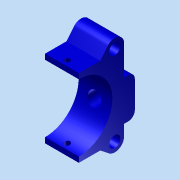
# Autodesk Inventor part: Axle Housing - Front - Custom
Saved by Autodesk Inventor 2012 (Build 160160000, 160)
## iProperties
Created: 2011-09-22
Part Number: Axle Housing - Front - Custom
Document SubType Name: Modeling
Designer: dgitz
Density: 1 g/cm^3
Material: Default
Author: dgitz
Autodesk Inventor part; units mm, degrees
ref_plane "YZ Plane" through (0, 0, 0) normal (1, 0, 0) x (0, 1, 0)
ref_plane "XZ Plane" through (0, 0, 0) normal (0, 1, 0) x (-1, 0, 0)
ref_plane "XY Plane" through (0, 0, 0) normal (0, 0, 1) x (1, 0, 0)
sketch "Sketch2" plane through (0, 0, 0) normal (1, 0, 0) x (0, 1, 0)
  circle A0 centre (100.6118, 121.1829) radius 2.667
  circle A1 centre (62.5118, 121.1829) radius 2.667
  line L0 (100.6118, 121.1829) -> (62.5118, 121.1829) construction
  arc A2 (100.6118, 116.7379) -> (103.3814, 124.6597) centre (100.6118, 121.1829) ccw
  arc A3 (59.0351, 123.9525) -> (62.5118, 116.7379) centre (62.5118, 121.1829) ccw
  line L1 (100.6118, 116.7379) -> (86.6418, 116.7379)
  line L2 (62.5118, 116.7379) -> (67.5918, 116.7379)
  line L3 (67.5918, 116.7379) -> (67.5918, 114.8329)
  line L4 (70.7668, 111.6579) -> (83.4668, 111.6579)
  line L5 (86.6418, 114.8329) -> (86.6418, 116.7379)
  arc A4 (64.8377, 138.2082) -> (96.5877, 138.2082) centre (80.7127, 138.2082) ccw
  line L6 (77.1168, 111.6579) -> (77.1168, 163.1454) construction
  line L7 (99.1277, 138.2082) -> (96.5877, 138.2082)
  line L8 (64.8377, 138.2082) -> (62.2977, 138.2082)
  line L9 (99.1277, 138.2082) -> (99.1277, 128.0482)
  line L10 (99.1277, 128.0482) -> (103.3814, 124.6597)
  line L11 (62.2977, 138.2082) -> (62.2977, 128.0482)
  line L12 (62.2977, 128.0482) -> (59.0351, 123.9525)
  line L13 (99.1277, 128.0482) -> (62.2977, 128.0482) construction
  arc A5 (83.4668, 111.6579) -> (86.6418, 114.8329) centre (83.4668, 114.8329) ccw
  arc A6 (67.5918, 114.8329) -> (70.7668, 111.6579) centre (70.7668, 114.8329) ccw
  point P0 (0, 0)
  point P1 (67.5918, 111.6579)
  point P2 (86.6418, 111.6579)
  dimension "d0" = 5.334
  dimension "d1" = 5.334
  dimension "d2" = 38.1
  dimension "d3" = 8.89
  dimension "d4" = 8.89
  dimension "d7" = 31.75
  dimension "d8" = 9.525
  dimension "d9" = 13.97
  dimension "d10" = 5.08
  dimension "d11" = 2.54
  dimension "d12" = 2.54
  dimension "d13" = 10.16
  dimension "d24" = 3.175
  constraints: 28 end point, 10 point on circle, 8 perpendicular, 8 tangent, 7 centre point, 5 point on line, 2 coincident, 2 horizontal, 2 vertical, 1 collinear, 1 equal radius, 1 midpoint, 1 parallel
  measures "d0" diameter of A0
  measures "d1" diameter of A1
  measures "d2" distance of L0.end L0.start
  measures "d3" diameter of A2
  measures "d4" diameter of A3
  measures "d7" diameter of A4
  measures "d8" distance from line of L4 L0.start
  measures "d9" distance from line of L5 L0.start
  measures "d10" distance from line of L3 L0.end
  measures "d11" distance of L7.end L7.start
  measures "d12" distance of L8.start L8.end
  measures "d13" distance from line of L9.end L7
  measures "d24" radius of A5
extrude "Extrusion1" add sketch "Sketch2" along normal mid plane 16.002
sketch "Sketch3" plane through (-8.001, 99.1277, 128.0482) normal (0, 1, 0) x (1, 0, 0)
  line L0 (0, 0) -> (0, -10.16) projected
  line L1 (0, -10.16) -> (16.002, -10.16) projected
  circle A0 centre (8.001, -7.62) radius 1.27
  point P0 (8.001, 128.0482)
  dimension "d16" = 2.54
  dimension "d17" = 8.001
  dimension "d18" = 2.54
  constraints: 1 centre point
  measures "d16" diameter of A0
  measures "d17" distance from line of A0.centre L0
  measures "d18" distance from line of A0.centre L1
extrude "Extrusion2" cut sketch "Sketch3" against normal up to surface (36.83 mm away)
sketch "Sketch6" plane through (8.001, 70.7668, 111.6579) normal (0, 0, -1) x (-1, 0, 0)
  circle A0 centre (8.001, 6.35) radius 3.175
  line L0 (0, 0) -> (16.002, 12.7) construction
  point P0 (8.001, -70.7668)
  dimension "d25" = 6.35
  constraints: 2 end point, 1 centre point, 1 coincident, 1 midpoint
  measures "d25" diameter of A0
extrude "Extrusion4" cut sketch "Sketch6" against normal blind 25.4
body "Solid1"
